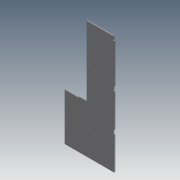
# Autodesk Inventor part: it side
Saved by Autodesk Inventor 2011 (Build 150239000, 239)
## iProperties
Created: 2011-09-03
Part Number: it side
Document SubType Name: Modeling
Designer: Matthew
Density: 1 g/cm^3
Author: Matthew
Autodesk Inventor part; units mm, degrees
(part 1 of 2)
ref_plane "YZ Plane" through (0, 0, 0) normal (1, 0, 0) x (0, 1, 0)
ref_plane "XZ Plane" through (0, 0, 0) normal (0, 1, 0) x (-1, 0, 0)
ref_plane "XY Plane" through (0, 0, 0) normal (0, 0, 1) x (1, 0, 0)
sketch "Sketch1" plane through (0, 0, 0) normal (0, 0, 1) x (1, 0, 0)
  line L0 (-30.3746, 22.0684) -> (296.0154, 22.0684)
  line L1 (296.0154, 22.0684) -> (296.0154, -866.9316)
  line L2 (296.0154, -866.9316) -> (-30.3746, -866.9316)
  line L3 (-30.3746, -866.9316) -> (-30.3746, 22.0684)
  point P0 (0, 0)
  dimension "d0" = 326.39
  dimension "d1" = 889
  constraints: 8 end point, 2 parallel, 1 horizontal, 1 perpendicular
  measures "d0" distance of L1.end L2.end
  measures "d1" distance of L0.end L1.end
extrude "Extrusion1" add sketch "Sketch1" along normal blind 6.35
sketch "Sketch2" plane through (0, 0, 6.35) normal (0, 0, 1) x (1, 0, 0)
  line L0 (296.0154, 22.0684) -> (296.0154, -866.9316) projected
  line L1 (296.0154, 22.0684) -> (289.6654, 22.0684)
  line L2 (289.6654, 22.0684) -> (289.6654, -28.7316)
  line L3 (289.6654, -28.7316) -> (296.0154, -28.7316)
  line L4 (296.0154, -28.7316) -> (296.0154, 22.0684)
  line L5 (289.6654, -28.7316) -> (296.0154, -28.7316)
  line L6 (296.0154, -28.7316) -> (296.0154, -79.5316)
  line L7 (296.0154, -79.5316) -> (289.6654, -79.5316)
  line L8 (289.6654, -79.5316) -> (289.6654, -28.7316)
  line L9 (289.6654, -79.5316) -> (296.0154, -79.5316)
  line L10 (296.0154, -79.5316) -> (296.0154, -130.3316)
  line L11 (296.0154, -130.3316) -> (289.6654, -130.3316)
  line L12 (289.6654, -130.3316) -> (289.6654, -79.5316)
  line L13 (289.6654, -130.3316) -> (296.0154, -130.3316)
  line L14 (296.0154, -130.3316) -> (296.0154, -181.1316)
  line L15 (296.0154, -181.1316) -> (289.6654, -181.1316)
  line L16 (289.6654, -181.1316) -> (289.6654, -130.3316)
  line L17 (289.6654, -181.1316) -> (296.0154, -181.1316)
  line L18 (296.0154, -181.1316) -> (296.0154, -231.9316)
  line L19 (296.0154, -231.9316) -> (289.6654, -231.9316)
  line L20 (289.6654, -231.9316) -> (289.6654, -181.1316)
  line L21 (289.6654, -231.9316) -> (296.0154, -231.9316)
  line L22 (296.0154, -231.9316) -> (296.0154, -282.7316)
  line L23 (296.0154, -282.7316) -> (289.6654, -282.7316)
  line L24 (289.6654, -282.7316) -> (289.6654, -231.9316)
  line L25 (289.6654, -282.7316) -> (296.0154, -282.7316)
  line L26 (296.0154, -282.7316) -> (296.0154, -333.5316)
  line L27 (296.0154, -333.5316) -> (289.6654, -333.5316)
  line L28 (289.6654, -333.5316) -> (289.6654, -282.7316)
  line L29 (289.6654, -333.5316) -> (296.0154, -333.5316)
  line L30 (296.0154, -333.5316) -> (296.0154, -384.3316)
  line L31 (296.0154, -384.3316) -> (289.6654, -384.3316)
  line L32 (289.6654, -384.3316) -> (289.6654, -333.5316)
  line L33 (289.6654, -384.3316) -> (296.0154, -384.3316)
  line L34 (296.0154, -384.3316) -> (296.0154, -435.1316)
  line L35 (296.0154, -435.1316) -> (289.6654, -435.1316)
  line L36 (289.6654, -435.1316) -> (289.6654, -384.3316)
  line L37 (289.6654, -435.1316) -> (296.0154, -435.1316)
  line L38 (296.0154, -435.1316) -> (296.0154, -485.9316)
  line L39 (296.0154, -485.9316) -> (289.6654, -485.9316)
  line L40 (289.6654, -485.9316) -> (289.6654, -435.1316)
  line L41 (289.6654, -485.9316) -> (296.0154, -485.9316)
  line L42 (296.0154, -485.9316) -> (296.0154, -536.7316)
  line L43 (296.0154, -536.7316) -> (289.6654, -536.7316)
  line L44 (289.6654, -536.7316) -> (289.6654, -485.9316)
  line L45 (289.6654, -536.7316) -> (296.0154, -536.7316)
  line L46 (296.0154, -536.7316) -> (296.0154, -587.5316)
  line L47 (296.0154, -587.5316) -> (289.6654, -587.5316)
  line L48 (289.6654, -587.5316) -> (289.6654, -536.7316)
  line L49 (289.6654, -587.5316) -> (296.0154, -587.5316)
  line L50 (296.0154, -587.5316) -> (296.0154, -638.3316)
  line L51 (296.0154, -638.3316) -> (289.6654, -638.3316)
  line L52 (289.6654, -638.3316) -> (289.6654, -587.5316)
  line L53 (289.6654, -638.3316) -> (296.0154, -638.3316)
  line L54 (296.0154, -638.3316) -> (296.0154, -689.1316)
  line L55 (296.0154, -689.1316) -> (289.6654, -689.1316)
  line L56 (289.6654, -689.1316) -> (289.6654, -638.3316)
  line L57 (289.6654, -689.1316) -> (296.0154, -689.1316)
  line L58 (296.0154, -689.1316) -> (296.0154, -739.9316)
  line L59 (296.0154, -739.9316) -> (289.6654, -739.9316)
  line L60 (289.6654, -739.9316) -> (289.6654, -689.1316)
  line L61 (289.6654, -739.9316) -> (296.0154, -739.9316)
  line L62 (296.0154, -739.9316) -> (296.0154, -790.7316)
  line L63 (296.0154, -790.7316) -> (289.6654, -790.7316)
  line L64 (289.6654, -790.7316) -> (289.6654, -739.9316)
  line L65 (289.6654, -790.7316) -> (296.0154, -790.7316)
  line L66 (296.0154, -790.7316) -> (296.0154, -841.5316)
  line L67 (296.0154, -841.5316) -> (289.6654, -841.5316)
  line L68 (289.6654, -841.5316) -> (289.6654, -790.7316)
  line L69 (289.6654, -841.5316) -> (296.0154, -841.5316)
  line L70 (296.0154, -841.5316) -> (296.0154, -866.9316)
  line L71 (296.0154, -866.9316) -> (289.6654, -866.9316)
  line L72 (289.6654, -866.9316) -> (289.6654, -841.5316)
  point P0 (0, 0)
  dimension "d4" = 6.35
  dimension "d5" = 50.8
  dimension "d6" = 50.8
  dimension "d7" = 50.8
  dimension "d8" = 50.8
  dimension "d9" = 50.8
  dimension "d10" = 50.8
  dimension "d11" = 50.8
  dimension "d12" = 50.8
  dimension "d13" = 50.8
  dimension "d14" = 50.8
  dimension "d15" = 50.8
  dimension "d16" = 50.8
  dimension "d17" = 50.8
  dimension "d18" = 50.8
  dimension "d19" = 50.8
  dimension "d20" = 50.8
  dimension "d21" = 50.8
  constraints: 144 end point, 36 parallel, 18 horizontal, 18 perpendicular, 17 other
  measures "d4" distance of L3.end L2.end
  measures "d5" distance of L2.end L1.end
  measures "d6" distance of L5.end L6.end
  measures "d7" distance of L9.end L10.end
  measures "d8" distance of L13.end L14.end
  measures "d9" distance of L17.end L18.end
  measures "d10" distance of L21.end L22.end
  measures "d11" distance of L25.end L26.end
  measures "d12" distance of L29.end L30.end
  measures "d13" distance of L33.end L34.end
  measures "d14" distance of L37.end L38.end
  measures "d15" distance of L41.end L42.end
  measures "d16" distance of L45.end L46.end
  measures "d17" distance of L49.end L50.end
  measures "d18" distance of L53.end L54.end
  measures "d19" distance of L57.end L58.end
  measures "d20" distance of L61.end L62.end
  measures "d21" distance of L65.end L66.end
extrude "Extrusion2" cut sketch "Sketch2" against normal blind 6.35 contours L0 L3 L2 L1 | L0 L11 L12 L7 | L0 L19 L20 L15 | L0 L27 L28 L23 | L0 L35 L36 L31 | L0 L43 L44 L39 | L0 L51 L52 L47 | L0 L59 L60 L55 | L0 L67 L68 L63 | L0 L71 L72 L67
sketch "Sketch3" plane through (0, 0, 6.35) normal (0, 0, 1) x (1, 0, 0)
  line L0 (-30.3746, -866.9316) -> (-30.3746, 22.0684) projected
  line L1 (289.6654, -866.9316) -> (-30.3746, -866.9316) projected
  line L2 (-30.3746, 22.0684) -> (-24.0246, 22.0684)
  line L3 (-24.0246, 22.0684) -> (-24.0246, -28.7316)
  line L4 (-24.0246, -28.7316) -> (-30.3746, -28.7316)
  line L5 (-30.3746, -28.7316) -> (-30.3746, 22.0684)
  line L6 (-30.3746, -28.7316) -> (-24.0246, -28.7316)
  line L7 (-24.0246, -28.7316) -> (-24.0246, -79.5316)
  line L8 (-24.0246, -79.5316) -> (-30.3746, -79.5316)
  line L9 (-30.3746, -79.5316) -> (-30.3746, -28.7316)
  line L10 (-24.0246, -79.5316) -> (-30.3746, -79.5316)
  line L11 (-30.3746, -79.5316) -> (-30.3746, -130.3316)
  line L12 (-30.3746, -130.3316) -> (-24.0246, -130.3316)
  line L13 (-24.0246, -130.3316) -> (-24.0246, -79.5316)
  line L14 (-24.0246, -130.3316) -> (-30.3746, -130.3316)
  line L15 (-30.3746, -130.3316) -> (-30.3746, -181.1316)
  line L16 (-30.3746, -181.1316) -> (-24.0246, -181.1316)
  line L17 (-24.0246, -181.1316) -> (-24.0246, -130.3316)
  line L18 (-30.3746, -181.1316) -> (-24.0246, -181.1316)
  line L19 (-24.0246, -181.1316) -> (-24.0246, -231.9316)
  line L20 (-24.0246, -231.9316) -> (-30.3746, -231.9316)
  line L21 (-30.3746, -231.9316) -> (-30.3746, -181.1316)
  line L22 (-24.0246, -231.9316) -> (-30.3746, -231.9316)
  line L23 (-30.3746, -231.9316) -> (-30.3746, -282.7316)
  line L24 (-30.3746, -282.7316) -> (-24.0246, -282.7316)
  line L25 (-24.0246, -282.7316) -> (-24.0246, -231.9316)
  line L26 (-30.3746, -282.7316) -> (-24.0246, -282.7316)
  line L27 (-24.0246, -282.7316) -> (-24.0246, -333.5316)
  line L28 (-24.0246, -333.5316) -> (-30.3746, -333.5316)
  line L29 (-30.3746, -333.5316) -> (-30.3746, -282.7316)
  line L30 (-24.0246, -333.5316) -> (-30.3746, -333.5316)
  line L31 (-30.3746, -333.5316) -> (-30.3746, -384.3316)
  line L32 (-30.3746, -384.3316) -> (-24.0246, -384.3316)
  line L33 (-24.0246, -384.3316) -> (-24.0246, -333.5316)
  line L34 (-30.3746, -384.3316) -> (-24.0246, -384.3316)
  line L35 (-24.0246, -384.3316) -> (-24.0246, -435.1316)
  line L36 (-24.0246, -435.1316) -> (-30.3746, -435.1316)
  line L37 (-30.3746, -435.1316) -> (-30.3746, -384.3316)
  line L38 (-24.0246, -435.1316) -> (-30.3746, -435.1316)
  line L39 (-30.3746, -435.1316) -> (-30.3746, -485.9316)
  line L40 (-30.3746, -485.9316) -> (-24.0246, -485.9316)
  line L41 (-24.0246, -485.9316) -> (-24.0246, -435.1316)
  line L42 (-30.3746, -485.9316) -> (-24.0246, -485.9316)
  line L43 (-24.0246, -485.9316) -> (-24.0246, -536.7316)
  line L44 (-24.0246, -536.7316) -> (-30.3746, -536.7316)
  line L45 (-30.3746, -536.7316) -> (-30.3746, -485.9316)
  line L46 (-24.0246, -536.7316) -> (-30.3746, -536.7316)
  line L47 (-30.3746, -536.7316) -> (-30.3746, -587.5316)
  line L48 (-30.3746, -587.5316) -> (-24.0246, -587.5316)
  line L49 (-24.0246, -587.5316) -> (-24.0246, -536.7316)
  line L50 (-30.3746, -587.5316) -> (-24.0246, -587.5316)
  line L51 (-24.0246, -587.5316) -> (-24.0246, -638.3316)
  line L52 (-24.0246, -638.3316) -> (-30.3746, -638.3316)
  line L53 (-30.3746, -638.3316) -> (-30.3746, -587.5316)
  line L54 (-24.0246, -638.3316) -> (-30.3746, -638.3316)
  line L55 (-30.3746, -638.3316) -> (-30.3746, -689.1316)
  line L56 (-30.3746, -689.1316) -> (-24.0246, -689.1316)
  line L57 (-24.0246, -689.1316) -> (-24.0246, -638.3316)
  line L58 (-30.3746, -689.1316) -> (-24.0246, -689.1316)
  line L59 (-24.0246, -689.1316) -> (-24.0246, -739.9316)
  line L60 (-24.0246, -739.9316) -> (-30.3746, -739.9316)
  line L61 (-30.3746, -739.9316) -> (-30.3746, -689.1316)
  line L62 (-30.3746, -739.9316) -> (-24.0246, -739.9316)
  line L63 (-24.0246, -739.9316) -> (-24.0246, -790.7316)
  line L64 (-24.0246, -790.7316) -> (-30.3746, -790.7316)
  line L65 (-30.3746, -790.7316) -> (-30.3746, -739.9316)
  line L66 (-30.3746, -790.7316) -> (-24.0246, -790.7316)
  line L67 (-24.0246, -790.7316) -> (-24.0246, -866.9316)
  line L68 (-24.0246, -866.9316) -> (-30.3746, -866.9316)
  line L69 (-30.3746, -866.9316) -> (-30.3746, -790.7316)
  point P0 (0, 0)
  dimension "d24" = 6.35
  constraints: 136 end point, 34 parallel, 17 horizontal, 17 perpendicular, 1 point on line, 8 other
  measures "d24" distance of L3.end L4.end
extrude "Extrusion3" cut sketch "Sketch3" against normal blind 6.35 contours L0 L64 L67 L1 | L0 L56 L59 L60 | L0 L48 L51 L52 | L0 L40 L43 L44 | L0 L32 L35 L36 | L0 L24 L27 L28 | L0 L16 L19 L20 | L0 L8 L13 L12 | L0 L2 L3 L4
sketch "Sketch4" plane through (0, 0, 6.35) normal (0, 0, 1) x (1, 0, 0)
  line L0 (-24.0246, 22.0684) -> (132.8204, 22.0684)
  line L1 (132.8204, 22.0684) -> (132.8204, 15.7184)
  line L2 (132.8204, 15.7184) -> (-24.0246, 15.7184)
  line L3 (-24.0246, 15.7184) -> (-24.0246, 22.0684)
  line L4 (132.8204, 22.0684) -> (158.2204, 22.0684)
  line L5 (158.2204, 22.0684) -> (158.2204, 15.7184)
  line L6 (158.2204, 15.7184) -> (132.8204, 15.7184)
  line L7 (132.8204, 15.7184) -> (132.8204, 22.0684)
  line L8 (158.2204, 22.0684) -> (209.0204, 22.0684)
  line L9 (209.0204, 22.0684) -> (209.0204, 15.7184)
  line L10 (209.0204, 15.7184) -> (158.2204, 15.7184)
  line L11 (158.2204, 15.7184) -> (158.2204, 22.0684)
  line L12 (209.0204, 22.0684) -> (259.8204, 22.0684)
  line L13 (259.8204, 22.0684) -> (259.8204, 15.7184)
  line L14 (259.8204, 15.7184) -> (209.0204, 15.7184)
  line L15 (209.0204, 15.7184) -> (209.0204, 22.0684)
  line L16 (132.8204, 22.0684) -> (107.4204, 22.0684)
  line L17 (107.4204, 22.0684) -> (107.4204, 15.7184)
  line L18 (107.4204, 15.7184) -> (132.8204, 15.7184)
  line L19 (132.8204, 15.7184) -> (132.8204, 22.0684)
  line L20 (107.4204, 22.0684) -> (56.6204, 22.0684)
  line L21 (56.6204, 22.0684) -> (56.6204, 15.7184)
  line L22 (56.6204, 15.7184) -> (107.4204, 15.7184)
  line L23 (107.4204, 15.7184) -> (107.4204, 22.0684)
  line L24 (56.6204, 22.0684) -> (5.8204, 22.0684)
  line L25 (5.8204, 22.0684) -> (5.8204, 15.7184)
  line L26 (5.8204, 15.7184) -> (56.6204, 15.7184)
  line L27 (56.6204, 15.7184) -> (56.6204, 22.0684)
  point P0 (0, 0)
  dimension "d27" = 156.845
  dimension "d28" = 6.35
  dimension "d29" = 25.4
  dimension "d30" = 50.8
  dimension "d31" = 50.8
  dimension "d32" = 25.4
  dimension "d33" = 50.8
  dimension "d34" = 50.8
  constraints: 56 end point, 14 parallel, 7 horizontal, 7 perpendicular, 3 point on line
  measures "d27" distance of L1.end L2.end
  measures "d28" distance of L0.end L1.end
  measures "d29" distance of L5.end L6.end
  measures "d30" distance of L9.end L10.end
  measures "d31" distance of L13.end L14.end
  measures "d32" distance of L18.end L17.end
  measures "d33" distance of L22.end L21.end
  measures "d34" distance of L26.end L25.end
extrude "Extrusion4" add sketch "Sketch4" along normal blind 6.35 contours L0 L21 L2 L25 | L0 L1 L2 L17 | L4 L5 L6 L1 | L12 L13 L14 L9
sketch "Sketch5" plane through (0, 0, 12.7) normal (0, 0, 1) x (1, 0, 0)
  line L0 (5.8204, 15.7184) -> (5.8204, 22.0684) projected
  line L1 (56.6204, 15.7184) -> (5.8204, 15.7184) projected
  line L2 (56.6204, 22.0684) -> (56.6204, 15.7184) projected
  line L3 (5.8204, 22.0684) -> (56.6204, 22.0684) projected
  point P0 (0, 0)
extrude "Extrusion5" cut sketch "Sketch5" against normal blind 25.4
sketch "Sketch6" plane through (0, 0, 12.7) normal (0, 0, 1) x (1, 0, 0)
  line L0 (107.4204, 22.0684) -> (158.2204, 22.0684) projected
  line L1 (107.4204, 15.7184) -> (107.4204, 22.0684) projected
  line L2 (158.2204, 15.7184) -> (107.4204, 15.7184) projected
  line L3 (158.2204, 22.0684) -> (158.2204, 15.7184) projected
  point P0 (0, 0)
extrude "Extrusion6" cut sketch "Sketch6" against normal blind 25.4
sketch "Sketch7" plane through (0, 0, 12.7) normal (0, 0, 1) x (1, 0, 0)
  line L0 (209.0204, 22.0684) -> (259.8204, 22.0684) projected
  line L1 (209.0204, 15.7184) -> (209.0204, 22.0684) projected
  line L2 (259.8204, 15.7184) -> (209.0204, 15.7184) projected
  line L3 (259.8204, 22.0684) -> (259.8204, 15.7184) projected
  point P0 (0, 0)
extrude "Extrusion7" cut sketch "Sketch7" against normal blind 25.4
sketch "Sketch8" plane through (0, 0, 6.35) normal (0, 0, 1) x (1, 0, 0)
  line L0 (289.6654, -866.9316) -> (-24.0246, -866.9316) projected
  line L1 (-24.0246, -866.9316) -> (5.8204, -866.9316)
  line L2 (5.8204, -866.9316) -> (5.8204, -860.5816)
  line L3 (5.8204, -860.5816) -> (-24.0246, -860.5816)
  line L4 (-24.0246, -860.5816) -> (-24.0246, -866.9316)
  line L5 (5.8204, -860.5816) -> (56.6204, -860.5816)
  line L6 (56.6204, -860.5816) -> (56.6204, -866.9316)
  line L7 (56.6204, -866.9316) -> (5.8204, -866.9316)
  line L8 (5.8204, -866.9316) -> (5.8204, -860.5816)
  line L9 (56.6204, -860.5816) -> (107.4204, -860.5816)
  line L10 (107.4204, -860.5816) -> (107.4204, -866.9316)
  line L11 (107.4204, -866.9316) -> (56.6204, -866.9316)
  line L12 (56.6204, -866.9316) -> (56.6204, -860.5816)
  line L13 (107.4204, -860.5816) -> (158.2204, -860.5816)
  line L14 (158.2204, -860.5816) -> (158.2204, -866.9316)
  line L15 (158.2204, -866.9316) -> (107.4204, -866.9316)
  line L16 (107.4204, -866.9316) -> (107.4204, -860.5816)
  line L17 (158.2204, -860.5816) -> (209.0204, -860.5816)
  line L18 (209.0204, -860.5816) -> (209.0204, -866.9316)
  line L19 (209.0204, -866.9316) -> (158.2204, -866.9316)
  line L20 (158.2204, -866.9316) -> (158.2204, -860.5816)
  line L21 (209.0204, -860.5816) -> (259.8204, -860.5816)
  line L22 (259.8204, -860.5816) -> (259.8204, -866.9316)
  line L23 (259.8204, -866.9316) -> (209.0204, -866.9316)
  line L24 (209.0204, -866.9316) -> (209.0204, -860.5816)
  point P0 (0, 0)
  dimension "d43" = 6.35
  constraints: 48 end point, 12 parallel, 6 horizontal, 6 perpendicular, 5 point on line
  measures "d43" distance of L2.end L1.end
extrude "Extrusion8" cut sketch "Sketch8" against normal blind 25.4 contours L0 L18 L21 L22 | L0 L10 L13 L14 | L0 L2 L5 L6
sketch "Sketch9" plane through (0, 0, 0) normal (0, 0, -1) x (-1, 0, 0)
  line L0 (-289.6654, -866.9316) -> (-276.9654, -866.9316)
  line L1 (-276.9654, -866.9316) -> (-276.9654, -822.4816)
  line L2 (-276.9654, -822.4816) -> (-289.6654, -822.4816)
  line L3 (-289.6654, -822.4816) -> (-289.6654, -866.9316)
  line L4 (24.0246, -866.9316) -> (11.3246, -866.9316)
  line L5 (11.3246, -866.9316) -> (11.3246, -822.4816)
  line L6 (11.3246, -822.4816) -> (24.0246, -822.4816)
  line L7 (24.0246, -822.4816) -> (24.0246, -866.9316)
  circle A0 centre (-276.9654, -822.4816) radius 1.9812
  circle A1 centre (11.3246, -822.4816) radius 1.9812
  point P0 (0, 0)
  dimension "d46" = 12.7
  dimension "d47" = 44.45
  dimension "d48" = 12.7
  dimension "d49" = 44.45
  dimension "d50" = 3.9624
  dimension "d51" = 3.9624
  constraints: 16 end point, 4 parallel, 2 centre point, 2 coincident, 2 horizontal, 2 perpendicular
  measures "d46" distance of L2.end L1.end
  measures "d47" distance of L1.end L0.end
  measures "d48" distance of L5.end L6.end
  measures "d49" distance of L4.end L5.end
  measures "d50" diameter of A0
  measures "d51" diameter of A1
extrude "Extrusion9" cut sketch "Sketch9" against normal blind 25.4 contours A0 L2 L1 | L1 L2 A0 | A1 L6 L5 | L5 L6 A1
sketch "Sketch10" plane through (0, 0, 0) normal (0, 0, -1) x (-1, 0, 0)
  circle A0 centre (-276.9654, -822.4816) radius 1.9812 projected
  point P0 (0, 0)
extrude "Extrusion10" add sketch "Sketch10" against normal blind 6.35
sketch "Sketch11" plane through (0, 0, 0) normal (0, 0, -1) x (-1, 0, 0)
  circle A0 centre (11.3246, -822.4816) radius 1.9812 projected
  point P0 (0, 0)
extrude "Extrusion11" add sketch "Sketch11" against normal blind 6.35
sketch "Sketch12" plane through (0, 0, 0) normal (0, 0, -1) x (-1, 0, 0)
  line L0 (-56.6204, -866.9316) -> (-56.6204, -860.5816) projected
  line L1 (-56.6204, -860.5816) -> (-5.8204, -860.5816) projected
  line L2 (-5.8204, -860.5816) -> (-5.8204, -866.9316) projected
  line L3 (-5.8204, -866.9316) -> (24.0246, -866.9316) projected
  line L4 (24.0246, -866.9316) -> (24.0246, -790.7316) projected
  line L5 (24.0246, -790.7316) -> (30.3746, -790.7316) projected
  line L6 (30.3746, -790.7316) -> (30.3746, -739.9316) projected
  line L7 (30.3746, -739.9316) -> (24.0246, -739.9316) projected
  line L8 (24.0246, -739.9316) -> (24.0246, -689.1316) projected
  line L9 (24.0246, -689.1316) -> (30.3746, -689.1316) projected
  line L10 (30.3746, -689.1316) -> (30.3746, -638.3316) projected
  line L11 (30.3746, -638.3316) -> (24.0246, -638.3316) projected
  line L12 (24.0246, -638.3316) -> (24.0246, -587.5316) projected
  line L13 (24.0246, -587.5316) -> (30.3746, -587.5316) projected
  line L14 (30.3746, -587.5316) -> (30.3746, -536.7316) projected
  line L15 (30.3746, -536.7316) -> (24.0246, -536.7316) projected
  line L16 (24.0246, -536.7316) -> (24.0246, -485.9316) projected
  line L17 (24.0246, -485.9316) -> (30.3746, -485.9316) projected
  line L18 (30.3746, -485.9316) -> (30.3746, -435.1316) projected
  line L19 (30.3746, -435.1316) -> (24.0246, -435.1316) projected
  line L20 (24.0246, -435.1316) -> (24.0246, -384.3316) projected
  line L21 (24.0246, -384.3316) -> (30.3746, -384.3316) projected
  line L22 (30.3746, -384.3316) -> (30.3746, -333.5316) projected
  line L23 (30.3746, -333.5316) -> (24.0246, -333.5316) projected
  line L24 (24.0246, -333.5316) -> (24.0246, -282.7316) projected
  line L25 (24.0246, -282.7316) -> (30.3746, -282.7316) projected
  line L26 (30.3746, -282.7316) -> (30.3746, -231.9316) projected
  line L27 (30.3746, -231.9316) -> (24.0246, -231.9316) projected
  line L28 (24.0246, -231.9316) -> (24.0246, -181.1316) projected
  line L29 (24.0246, -181.1316) -> (30.3746, -181.1316) projected
  line L30 (30.3746, -181.1316) -> (30.3746, -130.3316) projected
  line L31 (30.3746, -130.3316) -> (24.0246, -130.3316) projected
  line L32 (24.0246, -130.3316) -> (24.0246, -79.5316) projected
  line L33 (24.0246, -79.5316) -> (30.3746, -79.5316) projected
  line L34 (30.3746, -79.5316) -> (30.3746, -28.7316) projected
  line L35 (30.3746, -28.7316) -> (24.0246, -28.7316) projected
  line L36 (24.0246, -28.7316) -> (24.0246, 22.0684) projected
  line L37 (24.0246, 22.0684) -> (-5.8204, 22.0684) projected
  line L38 (-5.8204, 22.0684) -> (-5.8204, 15.7184) projected
  line L39 (-5.8204, 15.7184) -> (-56.6204, 15.7184) projected
  line L40 (-56.6204, 15.7184) -> (-56.6204, 22.0684) projected
  line L41 (-56.6204, 22.0684) -> (-107.4204, 22.0684) projected
  line L42 (-107.4204, 22.0684) -> (-107.4204, 15.7184) projected
  line L43 (-107.4204, 15.7184) -> (-158.2204, 15.7184) projected
  line L44 (-158.2204, 15.7184) -> (-158.2204, 22.0684) projected
  line L45 (-158.2204, 22.0684) -> (-209.0204, 22.0684) projected
  line L46 (-209.0204, 22.0684) -> (-209.0204, 15.7184) projected
  line L47 (-209.0204, 15.7184) -> (-259.8204, 15.7184) projected
  line L48 (-259.8204, 15.7184) -> (-259.8204, 22.0684) projected
  line L49 (-259.8204, 22.0684) -> (-289.6654, 22.0684) projected
  line L50 (-289.6654, 22.0684) -> (-289.6654, -28.7316) projected
  line L51 (-289.6654, -28.7316) -> (-296.0154, -28.7316) projected
  line L52 (-296.0154, -28.7316) -> (-296.0154, -79.5316) projected
  line L53 (-296.0154, -79.5316) -> (-289.6654, -79.5316) projected
  line L54 (-289.6654, -79.5316) -> (-289.6654, -130.3316) projected
  line L55 (-289.6654, -130.3316) -> (-296.0154, -130.3316) projected
  line L56 (-296.0154, -130.3316) -> (-296.0154, -181.1316) projected
  line L57 (-296.0154, -181.1316) -> (-289.6654, -181.1316) projected
  line L58 (-289.6654, -181.1316) -> (-289.6654, -231.9316) projected
  line L59 (-289.6654, -231.9316) -> (-296.0154, -231.9316) projected
  line L60 (-296.0154, -231.9316) -> (-296.0154, -282.7316) projected
  line L61 (-296.0154, -282.7316) -> (-289.6654, -282.7316) projected
  line L62 (-289.6654, -282.7316) -> (-289.6654, -333.5316) projected
  line L63 (-289.6654, -333.5316) -> (-296.0154, -333.5316) projected
  line L64 (-296.0154, -333.5316) -> (-296.0154, -384.3316) projected
  line L65 (-296.0154, -384.3316) -> (-289.6654, -384.3316) projected
  line L66 (-289.6654, -384.3316) -> (-289.6654, -435.1316) projected
  line L67 (-289.6654, -435.1316) -> (-296.0154, -435.1316) projected
  line L68 (-296.0154, -435.1316) -> (-296.0154, -485.9316) projected
  line L69 (-296.0154, -485.9316) -> (-289.6654, -485.9316) projected
  line L70 (-289.6654, -485.9316) -> (-289.6654, -536.7316) projected
  line L71 (-289.6654, -536.7316) -> (-296.0154, -536.7316) projected
  line L72 (-296.0154, -536.7316) -> (-296.0154, -587.5316) projected
  line L73 (-296.0154, -587.5316) -> (-289.6654, -587.5316) projected
  line L74 (-289.6654, -587.5316) -> (-289.6654, -638.3316) projected
  line L75 (-289.6654, -638.3316) -> (-296.0154, -638.3316) projected
  line L76 (-296.0154, -638.3316) -> (-296.0154, -689.1316) projected
  line L77 (-296.0154, -689.1316) -> (-289.6654, -689.1316) projected
  line L78 (-289.6654, -689.1316) -> (-289.6654, -739.9316) projected
  line L79 (-289.6654, -739.9316) -> (-296.0154, -739.9316) projected
  line L80 (-296.0154, -739.9316) -> (-296.0154, -790.7316) projected
  line L81 (-296.0154, -790.7316) -> (-289.6654, -790.7316) projected
  line L82 (-289.6654, -790.7316) -> (-289.6654, -866.9316) projected
  line L83 (-289.6654, -866.9316) -> (-259.8204, -866.9316) projected
  line L84 (-259.8204, -866.9316) -> (-259.8204, -860.5816) projected
  line L85 (-259.8204, -860.5816) -> (-209.0204, -860.5816) projected
  line L86 (-209.0204, -860.5816) -> (-209.0204, -866.9316) projected
  line L87 (-209.0204, -866.9316) -> (-158.2204, -866.9316) projected
  line L88 (-158.2204, -866.9316) -> (-158.2204, -860.5816) projected
  line L89 (-158.2204, -860.5816) -> (-107.4204, -860.5816) projected
  line L90 (-107.4204, -860.5816) -> (-107.4204, -866.9316) projected
  line L91 (-107.4204, -866.9316) -> (-56.6204, -866.9316) projected
  point P0 (0, 0)
sketch "Sketch13" plane through (0, 0, 0) normal (0, 0, -1) x (-1, 0, 0)
  line L0 (-289.6654, -866.9316) -> (-283.3154, -866.9316)
  line L1 (-283.3154, -866.9316) -> (-283.3154, -822.4816)
  line L2 (-283.3154, -822.4816) -> (-289.6654, -822.4816)
  line L3 (-289.6654, -822.4816) -> (-289.6654, -866.9316)
  line L4 (24.0246, -866.9316) -> (17.6746, -866.9316)
  line L5 (17.6746, -866.9316) -> (17.6746, -822.4816)
  line L6 (17.6746, -822.4816) -> (24.0246, -822.4816)
  line L7 (24.0246, -822.4816) -> (24.0246, -866.9316)
  circle A0 centre (-283.3154, -822.4816) radius 1.9812
  circle A1 centre (17.6746, -822.4816) radius 1.9812
  point P0 (0, 0)
  dimension "d58" = 6.35
  dimension "d59" = 44.45
  dimension "d60" = 6.35
  dimension "d61" = 3.9624
  dimension "d62" = 3.9624
  constraints: 16 end point, 4 parallel, 2 centre point, 2 coincident, 2 horizontal, 2 perpendicular
  measures "d58" distance of L2.end L1.end
  measures "d59" distance of L1.end L0.end
  measures "d60" distance of L5.end L6.end
  measures "d61" diameter of A0
  measures "d62" diameter of A1
extrude "Extrusion12" cut sketch "Sketch13" against normal blind 6.35 contours A0 L2 L1 | L1 L2 A0 | A1 L6 L5 | L5 L6 A1
sketch "Sketch14" plane through (0, 0, 0) normal (0, 0, -1) x (-1, 0, 0)
  line L0 (30.3746, -689.1316) -> (30.3746, -638.3316) projected
  line L1 (24.0246, -638.3316) -> (24.0246, -587.5316) projected
  line L2 (-289.6654, -587.5316) -> (-289.6654, -638.3316) projected
  line L3 (-289.6654, -638.3316) -> (-289.6654, -631.9816)
  line L4 (-289.6654, -631.9816) -> (-264.2654, -631.9816)
  line L5 (-264.2654, -631.9816) -> (-1.3754, -631.9816)
  line L6 (-1.3754, -631.9816) -> (-1.3754, -625.6316)
  line L7 (-1.3754, -625.6316) -> (-264.2654, -625.6316)
  line L8 (-264.2654, -625.6316) -> (-264.2654, -631.9816)
  point P0 (0, 0)
  dimension "d65" = 6.35
  dimension "d66" = 25.4
  dimension "d67" = 262.89
  dimension "d68" = 6.35
  constraints: 12 end point, 3 perpendicular, 2 parallel, 1 point on line
  measures "d65" distance of L2.end L3.end
  measures "d66" distance of L3.end L4.end
  measures "d67" distance of L4.end L5.end
  measures "d68" distance of L5.end L6.end
extrude "Extrusion13" cut sketch "Sketch14" against normal blind 25.4
sketch "Sketch15" plane through (0, 0, 0) normal (0, 0, -1) x (-1, 0, 0)
  line L0 (-1.3754, -625.6316) -> (-1.3754, -631.9816) projected
  line L1 (-1.3754, -631.9816) -> (-264.2654, -631.9816) projected
  line L2 (-264.2654, -631.9816) -> (-264.2654, -625.6316) projected
  line L3 (-264.2654, -625.6316) -> (-1.3754, -625.6316) projected
  point P0 (0, 0)
extrude "Extrusion14" add sketch "Sketch15" against normal blind 6.35
sketch "Sketch16" plane through (0, 0, 0) normal (0, 0, -1) x (-1, 0, 0)
  line L0 (-56.6204, -866.9316) -> (-56.6204, -860.5816) projected
  line L1 (-56.6204, -860.5816) -> (-5.8204, -860.5816) projected
  line L2 (-5.8204, -860.5816) -> (-5.8204, -866.9316) projected
  line L3 (-5.8204, -866.9316) -> (24.0246, -866.9316) projected
  line L4 (24.0246, -866.9316) -> (24.0246, -790.7316) projected
  line L5 (24.0246, -790.7316) -> (30.3746, -790.7316) projected
  line L6 (30.3746, -790.7316) -> (30.3746, -739.9316) projected
  line L7 (30.3746, -739.9316) -> (24.0246, -739.9316) projected
  line L8 (24.0246, -739.9316) -> (24.0246, -689.1316) projected
  line L9 (24.0246, -689.1316) -> (30.3746, -689.1316) projected
  line L10 (30.3746, -689.1316) -> (30.3746, -638.3316) projected
  line L11 (30.3746, -638.3316) -> (24.0246, -638.3316) projected
  line L12 (24.0246, -638.3316) -> (24.0246, -587.5316) projected
  line L13 (24.0246, -587.5316) -> (30.3746, -587.5316) projected
  line L14 (30.3746, -587.5316) -> (30.3746, -536.7316) projected
  line L15 (30.3746, -536.7316) -> (24.0246, -536.7316) projected
  line L16 (24.0246, -536.7316) -> (24.0246, -485.9316) projected
  line L17 (24.0246, -485.9316) -> (30.3746, -485.9316) projected
  line L18 (30.3746, -485.9316) -> (30.3746, -435.1316) projected
  line L19 (30.3746, -435.1316) -> (24.0246, -435.1316) projected
  line L20 (24.0246, -435.1316) -> (24.0246, -384.3316) projected
  line L21 (24.0246, -384.3316) -> (30.3746, -384.3316) projected
  line L22 (30.3746, -384.3316) -> (30.3746, -333.5316) projected
  line L23 (30.3746, -333.5316) -> (24.0246, -333.5316) projected
  line L24 (24.0246, -333.5316) -> (24.0246, -282.7316) projected
  line L25 (24.0246, -282.7316) -> (30.3746, -282.7316) projected
  line L26 (30.3746, -282.7316) -> (30.3746, -231.9316) projected
  line L27 (30.3746, -231.9316) -> (24.0246, -231.9316) projected
  line L28 (24.0246, -231.9316) -> (24.0246, -181.1316) projected
  line L29 (24.0246, -181.1316) -> (30.3746, -181.1316) projected
  line L30 (30.3746, -181.1316) -> (30.3746, -130.3316) projected
  line L31 (30.3746, -130.3316) -> (24.0246, -130.3316) projected
  line L32 (24.0246, -130.3316) -> (24.0246, -79.5316) projected
  line L33 (24.0246, -79.5316) -> (30.3746, -79.5316) projected
  line L34 (30.3746, -79.5316) -> (30.3746, -28.7316) projected
  line L35 (30.3746, -28.7316) -> (24.0246, -28.7316) projected
  line L36 (24.0246, -28.7316) -> (24.0246, 22.0684) projected
  line L37 (24.0246, 22.0684) -> (-5.8204, 22.0684) projected
  line L38 (-5.8204, 22.0684) -> (-5.8204, 15.7184) projected
  line L39 (-5.8204, 15.7184) -> (-56.6204, 15.7184) projected
  line L40 (-56.6204, 15.7184) -> (-56.6204, 22.0684) projected
  line L41 (-56.6204, 22.0684) -> (-107.4204, 22.0684) projected
  line L42 (-107.4204, 22.0684) -> (-107.4204, 15.7184) projected
  line L43 (-107.4204, 15.7184) -> (-158.2204, 15.7184) projected
  line L44 (-158.2204, 15.7184) -> (-158.2204, 22.0684) projected
  line L45 (-158.2204, 22.0684) -> (-209.0204, 22.0684) projected
  line L46 (-209.0204, 22.0684) -> (-209.0204, 15.7184) projected
  line L47 (-209.0204, 15.7184) -> (-259.8204, 15.7184) projected
  line L48 (-259.8204, 15.7184) -> (-259.8204, 22.0684) projected
  line L49 (-259.8204, 22.0684) -> (-289.6654, 22.0684) projected
  line L50 (-289.6654, 22.0684) -> (-289.6654, -28.7316) projected
  line L51 (-289.6654, -28.7316) -> (-296.0154, -28.7316) projected
  line L52 (-296.0154, -28.7316) -> (-296.0154, -79.5316) projected
  line L53 (-296.0154, -79.5316) -> (-289.6654, -79.5316) projected
  line L54 (-289.6654, -79.5316) -> (-289.6654, -130.3316) projected
  line L55 (-289.6654, -130.3316) -> (-296.0154, -130.3316) projected
  line L56 (-296.0154, -130.3316) -> (-296.0154, -181.1316) projected
  line L57 (-296.0154, -181.1316) -> (-289.6654, -181.1316) projected
  line L58 (-289.6654, -181.1316) -> (-289.6654, -231.9316) projected
  line L59 (-289.6654, -231.9316) -> (-296.0154, -231.9316) projected
  line L60 (-296.0154, -231.9316) -> (-296.0154, -282.7316) projected
  line L61 (-296.0154, -282.7316) -> (-289.6654, -282.7316) projected
  line L62 (-289.6654, -282.7316) -> (-289.6654, -333.5316) projected
  line L63 (-289.6654, -333.5316) -> (-296.0154, -333.5316) projected
  line L64 (-296.0154, -333.5316) -> (-296.0154, -384.3316) projected
  line L65 (-296.0154, -384.3316) -> (-289.6654, -384.3316) projected
  line L66 (-289.6654, -384.3316) -> (-289.6654, -435.1316) projected
  line L67 (-289.6654, -435.1316) -> (-296.0154, -435.1316) projected
  line L68 (-296.0154, -435.1316) -> (-296.0154, -485.9316) projected
  line L69 (-296.0154, -485.9316) -> (-289.6654, -485.9316) projected
  line L70 (-289.6654, -485.9316) -> (-289.6654, -536.7316) projected
  line L71 (-289.6654, -536.7316) -> (-296.0154, -536.7316) projected
  line L72 (-296.0154, -536.7316) -> (-296.0154, -587.5316) projected
  line L73 (-296.0154, -587.5316) -> (-289.6654, -587.5316) projected
  line L74 (-289.6654, -587.5316) -> (-289.6654, -638.3316) projected
  line L75 (-289.6654, -638.3316) -> (-296.0154, -638.3316) projected
  line L76 (-296.0154, -638.3316) -> (-296.0154, -689.1316) projected
  line L77 (-296.0154, -689.1316) -> (-289.6654, -689.1316) projected
  line L78 (-289.6654, -689.1316) -> (-289.6654, -739.9316) projected
  line L79 (-289.6654, -739.9316) -> (-296.0154, -739.9316) projected
  line L80 (-296.0154, -739.9316) -> (-296.0154, -790.7316) projected
  line L81 (-296.0154, -790.7316) -> (-289.6654, -790.7316) projected
  line L82 (-289.6654, -790.7316) -> (-289.6654, -866.9316) projected
  line L83 (-289.6654, -866.9316) -> (-259.8204, -866.9316) projected
  line L84 (-259.8204, -866.9316) -> (-259.8204, -860.5816) projected
  line L85 (-259.8204, -860.5816) -> (-209.0204, -860.5816) projected
  line L86 (-209.0204, -860.5816) -> (-209.0204, -866.9316) projected
  line L87 (-209.0204, -866.9316) -> (-158.2204, -866.9316) projected
  line L88 (-158.2204, -866.9316) -> (-158.2204, -860.5816) projected
  line L89 (-158.2204, -860.5816) -> (-107.4204, -860.5816) projected
  line L90 (-107.4204, -860.5816) -> (-107.4204, -866.9316) projected
  line L91 (-107.4204, -866.9316) -> (-56.6204, -866.9316) projected
  line L92 (-289.6654, -28.7316) -> (-289.6654, -790.7316)
  point P0 (0, 0)
  constraints: 2 end point, 1 collinear
extrude "Extrusion15" cut sketch "Sketch16" against normal blind 25.4 contours L81 L80 L79 L92 | L77 L76 L75 L92 | L73 L72 L71 L92 | L69 L68 L67 L92 | L65 L64 L63 L92 | L61 L60 L59 L92 | L57 L56 L55 L92 | L53 L52 L51 L92
sketch "Sketch17" plane through (0, 0, 0) normal (0, 0, -1) x (-1, 0, 0)
  line L0 (-289.6654, 22.0684) -> (-289.6654, -866.9316) projected
  line L1 (-289.6654, -866.9316) -> (-259.8204, -866.9316) projected
  line L2 (-259.8204, -866.9316) -> (-259.8204, -860.5816) projected
  line L3 (-259.8204, -860.5816) -> (-209.0204, -860.5816) projected
  line L4 (-209.0204, -860.5816) -> (-209.0204, -866.9316) projected
  line L5 (-209.0204, -866.9316) -> (-158.2204, -866.9316) projected
  line L6 (-158.2204, -866.9316) -> (-158.2204, -860.5816) projected
  line L7 (-158.2204, -860.5816) -> (-107.4204, -860.5816) projected
  line L8 (-107.4204, -860.5816) -> (-107.4204, -866.9316) projected
  line L9 (-107.4204, -866.9316) -> (-56.6204, -866.9316) projected
  line L10 (-56.6204, -866.9316) -> (-56.6204, -860.5816) projected
  line L11 (-56.6204, -860.5816) -> (-5.8204, -860.5816) projected
  line L12 (-5.8204, -860.5816) -> (-5.8204, -866.9316) projected
  line L13 (-5.8204, -866.9316) -> (24.0246, -866.9316) projected
  line L14 (24.0246, -866.9316) -> (24.0246, -790.7316) projected
  line L15 (24.0246, -790.7316) -> (30.3746, -790.7316) projected
  line L16 (30.3746, -790.7316) -> (30.3746, -739.9316) projected
  line L17 (30.3746, -739.9316) -> (24.0246, -739.9316) projected
  line L18 (24.0246, -739.9316) -> (24.0246, -689.1316) projected
  line L19 (24.0246, -689.1316) -> (30.3746, -689.1316) projected
  line L20 (30.3746, -689.1316) -> (30.3746, -638.3316) projected
  line L21 (30.3746, -638.3316) -> (24.0246, -638.3316) projected
  line L22 (24.0246, -638.3316) -> (24.0246, -587.5316) projected
  line L23 (24.0246, -587.5316) -> (30.3746, -587.5316) projected
  line L24 (30.3746, -587.5316) -> (30.3746, -536.7316) projected
  line L25 (30.3746, -536.7316) -> (24.0246, -536.7316) projected
  line L26 (24.0246, -536.7316) -> (24.0246, -485.9316) projected
  line L27 (24.0246, -485.9316) -> (30.3746, -485.9316) projected
  line L28 (30.3746, -485.9316) -> (30.3746, -435.1316) projected
  line L29 (30.3746, -435.1316) -> (24.0246, -435.1316) projected
  line L30 (24.0246, -435.1316) -> (24.0246, -384.3316) projected
  line L31 (24.0246, -384.3316) -> (30.3746, -384.3316) projected
  line L32 (30.3746, -384.3316) -> (30.3746, -333.5316) projected
  line L33 (30.3746, -333.5316) -> (24.0246, -333.5316) projected
  line L34 (24.0246, -333.5316) -> (24.0246, -282.7316) projected
  line L35 (24.0246, -282.7316) -> (30.3746, -282.7316) projected
  line L36 (30.3746, -282.7316) -> (30.3746, -231.9316) projected
  line L37 (30.3746, -231.9316) -> (24.0246, -231.9316) projected
  line L38 (24.0246, -231.9316) -> (24.0246, -181.1316) projected
  line L39 (24.0246, -181.1316) -> (30.3746, -181.1316) projected
  line L40 (30.3746, -181.1316) -> (30.3746, -130.3316) projected
  line L41 (30.3746, -130.3316) -> (24.0246, -130.3316) projected
  line L42 (24.0246, -130.3316) -> (24.0246, -79.5316) projected
  line L43 (24.0246, -79.5316) -> (30.3746, -79.5316) projected
  line L44 (30.3746, -79.5316) -> (30.3746, -28.7316) projected
  line L45 (30.3746, -28.7316) -> (24.0246, -28.7316) projected
  line L46 (24.0246, -28.7316) -> (24.0246, 22.0684) projected
  line L47 (24.0246, 22.0684) -> (-5.8204, 22.0684) projected
  line L48 (-5.8204, 22.0684) -> (-5.8204, 15.7184) projected
  line L49 (-5.8204, 15.7184) -> (-56.6204, 15.7184) projected
  line L50 (-56.6204, 15.7184) -> (-56.6204, 22.0684) projected
  line L51 (-56.6204, 22.0684) -> (-107.4204, 22.0684) projected
  line L52 (-107.4204, 22.0684) -> (-107.4204, 15.7184) projected
  line L53 (-107.4204, 15.7184) -> (-158.2204, 15.7184) projected
  line L54 (-158.2204, 15.7184) -> (-158.2204, 22.0684) projected
  line L55 (-158.2204, 22.0684) -> (-209.0204, 22.0684) projected
  line L56 (-209.0204, 22.0684) -> (-209.0204, 15.7184) projected
  line L57 (-209.0204, 15.7184) -> (-259.8204, 15.7184) projected
  line L58 (-259.8204, 15.7184) -> (-259.8204, 22.0684) projected
  line L59 (-259.8204, 22.0684) -> (-289.6654, 22.0684) projected
  line L60 (-289.6654, 15.7184) -> (24.0246, 15.7184)
  point P0 (0, 0)
  constraints: 2 end point, 2 point on line, 1 perpendicular
extrude "Extrusion16" cut sketch "Sketch17" against normal blind 25.4 contours L59 L58 L60 L0 | L56 L55 L54 L60 | L52 L51 L50 L60 | L48 L47 L46 L60
sketch "Sketch18" plane through (0, 0, 0) normal (0, 0, -1) x (-1, 0, 0)
  line L0 (24.0246, 15.7184) -> (-289.6654, 15.7184) projected
  line L1 (-289.6654, 15.7184) -> (-289.6654, -866.9316) projected
  line L2 (-289.6654, -866.9316) -> (-259.8204, -866.9316) projected
  line L3 (-259.8204, -866.9316) -> (-259.8204, -860.5816) projected
  line L4 (-259.8204, -860.5816) -> (-209.0204, -860.5816) projected
  line L5 (-209.0204, -860.5816) -> (-209.0204, -866.9316) projected
  line L6 (-209.0204, -866.9316) -> (-158.2204, -866.9316) projected
  line L7 (-158.2204, -866.9316) -> (-158.2204, -860.5816) projected
  line L8 (-158.2204, -860.5816) -> (-107.4204, -860.5816) projected
  line L9 (-107.4204, -860.5816) -> (-107.4204, -866.9316) projected
  line L10 (-107.4204, -866.9316) -> (-56.6204, -866.9316) projected
  line L11 (-56.6204, -866.9316) -> (-56.6204, -860.5816) projected
  line L12 (-56.6204, -860.5816) -> (-5.8204, -860.5816) projected
  line L13 (-5.8204, -860.5816) -> (-5.8204, -866.9316) projected
  line L14 (-5.8204, -866.9316) -> (24.0246, -866.9316) projected
  line L15 (24.0246, -866.9316) -> (24.0246, -790.7316) projected
  line L16 (24.0246, -790.7316) -> (30.3746, -790.7316) projected
  line L17 (30.3746, -790.7316) -> (30.3746, -739.9316) projected
  line L18 (30.3746, -739.9316) -> (24.0246, -739.9316) projected
  line L19 (24.0246, -739.9316) -> (24.0246, -689.1316) projected
  line L20 (24.0246, -689.1316) -> (30.3746, -689.1316) projected
  line L21 (30.3746, -689.1316) -> (30.3746, -638.3316) projected
  line L22 (30.3746, -638.3316) -> (24.0246, -638.3316) projected
  line L23 (24.0246, -638.3316) -> (24.0246, -587.5316) projected
  line L24 (24.0246, -587.5316) -> (30.3746, -587.5316) projected
  line L25 (30.3746, -587.5316) -> (30.3746, -536.7316) projected
  line L26 (30.3746, -536.7316) -> (24.0246, -536.7316) projected
  line L27 (24.0246, -536.7316) -> (24.0246, -485.9316) projected
  line L28 (24.0246, -485.9316) -> (30.3746, -485.9316) projected
  line L29 (30.3746, -485.9316) -> (30.3746, -435.1316) projected
  line L30 (30.3746, -435.1316) -> (24.0246, -435.1316) projected
  line L31 (24.0246, -435.1316) -> (24.0246, -384.3316) projected
  line L32 (24.0246, -384.3316) -> (30.3746, -384.3316) projected
  line L33 (30.3746, -384.3316) -> (30.3746, -333.5316) projected
  line L34 (30.3746, -333.5316) -> (24.0246, -333.5316) projected
  line L35 (24.0246, -333.5316) -> (24.0246, -282.7316) projected
  line L36 (24.0246, -282.7316) -> (30.3746, -282.7316) projected
  line L37 (30.3746, -282.7316) -> (30.3746, -231.9316) projected
  line L38 (30.3746, -231.9316) -> (24.0246, -231.9316) projected
  line L39 (24.0246, -231.9316) -> (24.0246, -181.1316) projected
  line L40 (24.0246, -181.1316) -> (30.3746, -181.1316) projected
  line L41 (30.3746, -181.1316) -> (30.3746, -130.3316) projected
  line L42 (30.3746, -130.3316) -> (24.0246, -130.3316) projected
  line L43 (24.0246, -130.3316) -> (24.0246, -79.5316) projected
  line L44 (24.0246, -79.5316) -> (30.3746, -79.5316) projected
  line L45 (30.3746, -79.5316) -> (30.3746, -28.7316) projected
  line L46 (30.3746, -28.7316) -> (24.0246, -28.7316) projected
  line L47 (24.0246, -28.7316) -> (24.0246, 15.7184) projected
  line L48 (24.0246, -28.7316) -> (24.0246, -790.7316)
  point P0 (0, 0)
  constraints: 2 end point, 1 collinear
extrude "Extrusion17" cut sketch "Sketch18" against normal blind 25.4 contours L46 L45 L44 L48 | L42 L41 L40 L48 | L38 L37 L36 L48 | L34 L33 L32 L48 | L30 L29 L28 L48 | L26 L25 L24 L48 | L22 L21 L20 L48 | L18 L17 L16 L48
sketch "Sketch19" plane through (0, 0, 0) normal (0, 0, -1) x (-1, 0, 0)
  line L0 (24.0246, -866.9316) -> (24.0246, 15.7184) projected
  line L1 (24.0246, 15.7184) -> (-289.6654, 15.7184) projected
  line L2 (-289.6654, 15.7184) -> (-289.6654, -866.9316) projected
  line L3 (-289.6654, -866.9316) -> (-259.8204, -866.9316) projected
  line L4 (-259.8204, -866.9316) -> (-259.8204, -860.5816) projected
  line L5 (-259.8204, -860.5816) -> (-209.0204, -860.5816) projected
  line L6 (-209.0204, -860.5816) -> (-209.0204, -866.9316) projected
  line L7 (-209.0204, -866.9316) -> (-158.2204, -866.9316) projected
  line L8 (-158.2204, -866.9316) -> (-158.2204, -860.5816) projected
  line L9 (-158.2204, -860.5816) -> (-107.4204, -860.5816) projected
  line L10 (-107.4204, -860.5816) -> (-107.4204, -866.9316) projected
  line L11 (-107.4204, -866.9316) -> (-56.6204, -866.9316) projected
  line L12 (-56.6204, -866.9316) -> (-56.6204, -860.5816) projected
  line L13 (-56.6204, -860.5816) -> (-5.8204, -860.5816) projected
  line L14 (-5.8204, -860.5816) -> (-5.8204, -866.9316) projected
  line L15 (-5.8204, -866.9316) -> (24.0246, -866.9316) projected
  line L16 (-259.8204, -866.9316) -> (-5.8204, -866.9316)
  point P0 (0, 0)
  constraints: 2 end point, 1 collinear
extrude "Extrusion18" add sketch "Sketch19" against normal blind 6.35 contours L16 L12 L13 L14 | L16 L8 L9 L10 | L4 L5 L6 L16
sketch "Sketch20" plane through (0, 0, 0) normal (0, 0, -1) x (-1, 0, 0)
  circle A0 centre (17.6746, -822.4816) radius 1.9812 projected
  circle A1 centre (-283.3154, -822.4816) radius 1.9812 projected
  point P0 (0, 0)
extrude "Extrusion19" add sketch "Sketch20" against normal blind 6.35
sketch "Sketch21" plane through (0, 0, 0) normal (0, 0, -1) x (-1, 0, 0)
  line L0 (24.0246, -866.9316) -> (24.0246, 15.7184) projected
  line L1 (24.0246, -866.9316) -> (24.0246, -555.7816)
  line L2 (24.0246, -555.7816) -> (-122.0254, -555.7816)
  line L3 (-122.0254, -555.7816) -> (-122.0254, -166.5437)
  line L4 (-122.0254, -166.5437) -> (24.0246, -166.5437)
  point P0 (0, 0)
  dimension "d83" = 311.15
  dimension "d84" = 146.05
  constraints: 8 end point, 2 perpendicular, 2 point on line, 1 parallel
  measures "d83" distance of L0.start L1.end
  measures "d84" distance of L1.end L2.end
extrude "Extrusion20" cut sketch "Sketch21" against normal blind 25.4
sketch "Sketch22" plane through (0, 0, 0) normal (0, 0, -1) x (-1, 0, 0)
  line L0 (24.0246, -166.5437) -> (24.0246, 15.7184) projected
  line L1 (24.0246, 15.7184) -> (-289.6654, 15.7184) projected
  line L2 (-289.6654, 15.7184) -> (-289.6654, -866.9316) projected
  line L3 (-289.6654, -866.9316) -> (-289.6654, -75.9756)
  line L4 (-289.6654, -75.9756) -> (-289.6654, -82.3256)
  line L5 (-289.6654, -82.3256) -> (24.0246, -82.3256)
  point P0 (0, 0)
  dimension "d87" = 790.956
  dimension "d88" = 6.35
  constraints: 6 end point, 3 point on line, 1 perpendicular
  measures "d87" distance of L2.end L3.end
  measures "d88" distance of L3.end L4.end
extrude "Extrusion21" cut sketch "Sketch22" against normal blind 25.4
sketch "Sketch23" plane through (0, 0, 0) normal (0, 0, -1) x (-1, 0, 0)
  line L0 (24.0246, -82.3256) -> (-289.6654, -82.3256) projected
  line L1 (-122.0254, -166.5437) -> (24.0246, -166.5437) projected
  line L2 (24.0246, -166.5437) -> (24.0246, -82.3256) projected
  line L3 (-122.0254, -166.5437) -> (-122.0254, -82.3256)
  point P0 (0, 0)
  constraints: 2 end point, 1 perpendicular, 1 point on line
extrude "Extrusion22" cut sketch "Sketch23" against normal blind 25.4
sketch "Sketch24" plane through (0, 0, 6.35) normal (0, 0, 1) x (1, 0, 0)
  line L0 (-24.0246, -555.7816) -> (122.0254, -555.7816)
  line L1 (122.0254, -555.7816) -> (122.0254, -562.1316)
  line L2 (122.0254, -562.1316) -> (-24.0246, -562.1316)
  line L3 (-24.0246, -562.1316) -> (-24.0246, -555.7816)
  point P0 (0, 0)
  dimension "d93" = 6.35
  constraints: 8 end point, 2 parallel, 1 horizontal, 1 perpendicular
  measures "d93" distance of L0.end L1.end
extrude "Extrusion23" cut sketch "Sketch24" against normal blind 25.4
sketch "Sketch25" plane through (0, 0, 6.35) normal (0, 0, 1) x (1, 0, 0)
  line L0 (122.0254, -82.3256) -> (122.0254, -562.1316) projected
  line L1 (-24.0246, -562.1316) -> (122.0254, -562.1316)
  line L2 (122.0254, -562.1316) -> (122.0254, -555.7816)
  line L3 (122.0254, -555.7816) -> (-24.0246, -555.7816)
  line L4 (-24.0246, -555.7816) -> (-24.0246, -562.1316)
  line L5 (122.0254, -555.7816) -> (115.9294, -555.7816)
  line L6 (115.9294, -555.7816) -> (115.9294, -82.3256)
  line L7 (115.9294, -82.3256) -> (122.0254, -82.3256)
  line L8 (122.0254, -82.3256) -> (122.0254, -555.7816)
  point P0 (0, 0)
  dimension "d96" = 6.35
  dimension "d97" = 6.096
  constraints: 16 end point, 4 parallel, 2 horizontal, 2 perpendicular, 1 point on line
  measures "d96" distance of L2.end L1.end
  measures "d97" distance of L6.end L7.end
extrude "Extrusion24" add sketch "Sketch25" against normal blind 6.35
sketch "Sketch26" plane through (0, 0, 0) normal (0, 0, -1) x (-1, 0, 0)
  line L0 (24.0246, -866.9316) -> (24.0246, -555.7816) projected
  line L1 (-115.9294, -555.7816) -> (24.0246, -555.7816)
  line L2 (24.0246, -555.7816) -> (24.0246, -562.1316)
  line L3 (24.0246, -562.1316) -> (-115.9294, -562.1316)
  line L4 (-115.9294, -562.1316) -> (-115.9294, -555.7816)
  point P0 (0, 0)
  dimension "d100" = 6.35
  constraints: 8 end point, 2 parallel, 1 horizontal, 1 perpendicular, 1 point on line
  measures "d100" distance of L1.end L2.end
extrude "Extrusion25" cut sketch "Sketch26" against normal blind 6.35
sketch "Sketch27" plane through (0, 0, 0) normal (0, 0, -1) x (-1, 0, 0)
  line L0 (-115.9294, -562.1316) -> (-115.9294, -82.3256) projected
  line L1 (-289.6654, -82.3256) -> (-115.9294, -82.3256)
  line L2 (-115.9294, -82.3256) -> (-115.9294, -88.6756)
  line L3 (-115.9294, -88.6756) -> (-289.6654, -88.6756)
  line L4 (-289.6654, -88.6756) -> (-289.6654, -82.3256)
  point P0 (0, 0)
  dimension "d103" = 6.35
  constraints: 8 end point, 2 parallel, 1 horizontal, 1 perpendicular, 1 point on line
  measures "d103" distance of L1.end L2.end
extrude "Extrusion26" cut sketch "Sketch27" against normal blind 6.35
sketch "Sketch28" plane through (0, 0, 6.35) normal (0, 0, 1) x (1, 0, 0)
  line L0 (115.9294, -562.1316) -> (-24.0246, -562.1316)
  line L1 (-24.0246, -562.1316) -> (-24.0246, -555.7816)
  line L2 (-24.0246, -555.7816) -> (115.9294, -555.7816)
  line L3 (115.9294, -555.7816) -> (115.9294, -562.1316)
  point P0 (0, 0)
  dimension "d106" = 6.35
  constraints: 8 end point, 2 parallel, 1 horizontal, 1 perpendicular
  measures "d106" distance of L0.end L1.end
extrude "Extrusion27" add sketch "Sketch28" against normal blind 6.35
sketch "Sketch29" plane through (0, 0, 0) normal (0, 0, -1) x (-1, 0, 0)
  line L0 (24.0246, -555.7816) -> (24.0246, -866.9316) projected
  line L1 (-115.9294, -555.7816) -> (24.0246, -555.7816)
  line L2 (24.0246, -555.7816) -> (24.0246, -562.1316)
  line L3 (24.0246, -562.1316) -> (-115.9294, -562.1316)
  line L4 (-115.9294, -562.1316) -> (-115.9294, -555.7816)
  point P0 (0, 0)
  dimension "d109" = 6.35
  constraints: 8 end point, 2 parallel, 1 horizontal, 1 perpendicular, 1 point on line
  measures "d109" distance of L1.end L2.end
extrude "Extrusion28" cut sketch "Sketch29" against normal blind 25.4
sketch "Sketch30" plane through (0, 0, 0) normal (0, 0, -1) x (-1, 0, 0)
  line L0 (24.0246, -562.1316) -> (-58.5254, -562.1316)
  line L1 (-58.5254, -562.1316) -> (-58.5254, -568.4816)
  line L2 (-58.5254, -568.4816) -> (24.0246, -568.4816)
  line L3 (24.0246, -568.4816) -> (24.0246, -562.1316)
  point P0 (0, 0)
  dimension "d112" = 82.55
  dimension "d113" = 6.35
  constraints: 8 end point, 2 parallel, 1 horizontal, 1 perpendicular
  measures "d112" distance of L2.end L1.end
  measures "d113" distance of L1.end L0.end
extrude "Extrusion29" cut sketch "Sketch30" against normal blind 25.4
sketch "Sketch31" plane through (0, 0, 6.35) normal (0, 0, 1) x (1, 0, 0)
  line L0 (289.6654, -866.9316) -> (289.6654, -88.6756) projected
  line L1 (115.9294, -88.6756) -> (289.6654, -88.6756)
  line L2 (289.6654, -88.6756) -> (289.6654, -107.7256)
  line L3 (289.6654, -107.7256) -> (115.9294, -107.7256)
  line L4 (115.9294, -107.7256) -> (115.9294, -88.6756)
  point P0 (0, 0)
  dimension "d116" = 19.05
  constraints: 8 end point, 2 parallel, 1 horizontal, 1 perpendicular, 1 point on line
  measures "d116" distance of L1.end L2.end
extrude "Extrusion30" cut sketch "Sketch31" against normal blind 25.4
sketch "Sketch32" plane through (0, 0, 6.35) normal (0, 0, 1) x (1, 0, 0)
  line L0 (289.6654, -866.9316) -> (289.6654, -107.7256) projected
  line L1 (289.6654, -866.9316) -> (289.6654, -625.6316)
  line L2 (289.6654, -625.6316) -> (289.6654, -631.9816)
  line L3 (289.6654, -631.9816) -> (289.6654, -644.6816)
  line L4 (289.6654, -644.6816) -> (283.3154, -644.6816)
  line L5 (283.3154, -644.6816) -> (283.3154, -631.9816)
  line L6 (283.3154, -631.9816) -> (289.6654, -631.9816)
  point P0 (0, 0)
  dimension "d119" = 241.3
  dimension "d120" = 6.35
  dimension "d121" = 12.7
  dimension "d122" = 6.35
  constraints: 12 end point, 3 point on line, 2 perpendicular, 1 parallel
  measures "d119" distance of L0.start L1.end
  measures "d120" distance of L1.end L2.end
  measures "d121" distance of L2.end L3.end
  measures "d122" distance of L3.end L4.end
extrude "Extrusion31" cut sketch "Sketch32" against normal blind 25.4
sketch "Sketch33" plane through (0, 0, 6.35) normal (0, 0, 1) x (1, 0, 0)
  line L0 (289.6654, -866.9316) -> (289.6654, -644.6816) projected
  line L1 (283.3154, -644.6816) -> (289.6654, -644.6816)
  line L2 (289.6654, -644.6816) -> (289.6654, -657.3816)
  line L3 (289.6654, -657.3816) -> (283.3154, -657.3816)
  line L4 (283.3154, -657.3816) -> (283.3154, -644.6816)
  point P0 (0, 0)
  dimension "d125" = 12.7
  constraints: 8 end point, 2 parallel, 1 horizontal, 1 perpendicular, 1 point on line
  measures "d125" distance of L1.end L2.end
extrude "Extrusion32" cut sketch "Sketch33" against normal blind 25.4
sketch "Sketch34" plane through (0, 0, 6.35) normal (0, 0, 1) x (1, 0, 0)
  line L0 (289.6654, -631.9816) -> (289.6654, -107.7256) projected
  line L1 (289.6654, -631.9816) -> (289.6654, -422.4316)
  line L2 (289.6654, -422.4316) -> (289.6654, -397.0316)
  line L3 (289.6654, -397.0316) -> (283.3154, -397.0316)
  line L4 (283.3154, -397.0316) -> (283.3154, -422.4316)
  line L5 (283.3154, -422.4316) -> (289.6654, -422.4316)
  line L6 (289.6654, -422.4316) -> (289.6654, -397.0316)
  point P0 (0, 0)
  dimension "d128" = 209.55
  dimension "d129" = 25.4
  dimension "d130" = 6.35
  constraints: 12 end point, 2 parallel, 2 point on line, 1 horizontal, 1 perpendicular
  measures "d128" distance of L0.start L1.end
  measures "d129" distance of L1.end L2.end
  measures "d130" distance of L5.end L4.end
extrude "Extrusion33" cut sketch "Sketch34" against normal blind 25.4